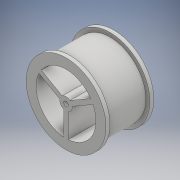
# Autodesk Inventor part: Wheel down
Saved by Autodesk Inventor 2018 (Build 220112000, 112)
## iProperties
Created: 2019-04-02
Part Number: Wheel down
Material: Типовые
Document SubType Name: Modeling
Designer: cosko
Density: 1 g/cm^3
Appearance: По умолчанию
Author: cosko
Autodesk Inventor part; units mm, degrees
ref_plane "YZ Plane" through (0, 0, 0) normal (1, 0, 0) x (0, 1, 0)
ref_plane "XZ Plane" through (0, 0, 0) normal (0, 1, 0) x (-1, 0, 0)
ref_plane "XY Plane" through (0, 0, 0) normal (0, 0, 1) x (1, 0, 0)
sketch "Эскиз1" plane through (0, 0, 0) normal (0, 0, 1) x (1, 0, 0)
  line L0 (0, 0) -> (15, 0)
  line L1 (15, 0) -> (15, 10)
  line L2 (15, 10) -> (15, -10)
  line L3 (15, 10) -> (18, 10)
  line L4 (18, 10) -> (18, -10)
  line L5 (18, -10) -> (15, -10)
  line L6 (15, -10) -> (15, 10)
  line L7 (15, 10) -> (20, 10)
  line L8 (20, 10) -> (20, 12)
  line L9 (20, 12) -> (15, 12)
  line L10 (15, 12) -> (15, 10)
  line L11 (15, -10) -> (20, -10)
  line L12 (20, -10) -> (20, -12)
  line L13 (20, -12) -> (15, -12)
  line L14 (15, -12) -> (15, -10)
  line L15 (0, 0) -> (0, 10)
  dimension "d0" = 15
  dimension "d1" = 10
  dimension "d2" = 20
  dimension "d3" = 3
  dimension "d4" = 5
  dimension "d5" = 2
  dimension "d6" = 5
  dimension "d7" = 2
  constraints: 32 end point, 6 parallel, 4 horizontal, 3 perpendicular, 2 vertical, 1 point on line
  measures "d0" distance of L0.start L0.end
  measures "d1" distance of L0.end L1.end
  measures "d2" distance of L1.end L2.end
  measures "d3" distance of L4.end L5.end
  measures "d4" distance of L9.end L8.end
  measures "d5" distance of L8.end L7.end
  measures "d6" distance of L12.end L13.end
  measures "d7" distance of L11.end L12.end
revolve "Вращение1" add sketch "Эскиз1" angle 360 about axis through (0, 0, 0) along (0, 1, 0)
sketch "Эскиз2" plane through (0, -12, 0) normal (0, -1, 0) x (1, 0, 0)
  circle A0 centre (0, 0) radius 1.15
  circle A1 centre (0, 0) radius 3.15
  circle A2 centre (0, 0) radius 15 projected
  line L0 (-1.15, 0) -> (1.15, 0)
  line L1 (1.15, 0) -> (1.15, -15.6419)
  line L2 (1.15, -15.6419) -> (-1.15, -15.6419)
  line L3 (-1.15, -15.6419) -> (-1.15, 0)
  line L4 (14.1213, 6.825) -> (0.575, -0.9959)
  line L5 (-0.575, 0.9959) -> (12.9713, 8.8169)
  line L6 (12.9713, 8.8169) -> (14.1213, 6.825)
  line L7 (0.575, -0.9959) -> (-0.575, 0.9959)
  line L8 (-12.9713, 8.8169) -> (0.575, 0.9959)
  line L9 (-0.575, -0.9959) -> (-14.1213, 6.825)
  line L10 (-14.1213, 6.825) -> (-12.9713, 8.8169)
  line L11 (0.575, 0.9959) -> (-0.575, -0.9959)
  dimension "d9" = 2.3
  dimension "d10" = 2
  dimension "d13" = 360
  constraints: 24 end point, 2 parallel, 1 centre point, 1 coincident, 1 horizontal, 1 horizontal alignment, 1 perpendicular, 27 other
extrude "Выдавливание1" add sketch "Эскиз2" against normal up to surface (24 mm away) contours L0 L11 A0 | L1 L4 A0 | A0 L7 L0 | A0 L8 L5 A1 L4 L1 | L11 L7 A0 | A0 L5 L8 | L4 L1 A1 L3 L9 A0 | A0 L11 L7 | L11 A0 L0 | L0 A0 L7 | L4 A1 L1 | A0 L3 L9 A1 L8 L5 | L8 A1 L5 | L9 L3 A0 | L1 A2 L3 A1 | A1 L5 A2 L4 | A1 L9 A2 L8 | L3 A1 L9 | L1 L2 L3 A2 | A2 L5 L6 L4 | A2 L9 L10 L8
extrude "Выдавливание2" cut sketch "Эскиз2" against normal up to surface (24 mm away) contours L0 L11 A0 | A0 L7 L0 | L11 L7 A0 | A0 L11 L7 | L11 A0 L0 | L0 A0 L7
